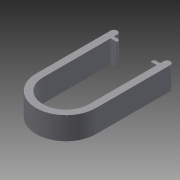
# Autodesk Inventor part: Pinza tapón tornillo
Saved by Autodesk Inventor 2014 (Build 180170000, 170)
## iProperties
Created: 2015-05-28
Part Number: Pinza tapón tornillo
Material: Generic
Document SubType Name: Modeling
Designer: Rubén
Density: 1 g/cm^3
Appearance: Default
Author: Rubén
Autodesk Inventor part; units mm, degrees
ref_plane "YZ Plane" through (0, 0, 0) normal (1, 0, 0) x (0, 1, 0)
ref_plane "XZ Plane" through (0, 0, 0) normal (0, 1, 0) x (-1, 0, 0)
ref_plane "XY Plane" through (0, 0, 0) normal (0, 0, 1) x (1, 0, 0)
sketch "Sketch1" plane through (0, 0, 0) normal (0, 1, 0) x (-1, 0, 0)
  line L0 (10.25, 0) -> (10.25, 30)
  arc A0 (10.25, 30) -> (0, 40.25) centre (0, 30) ccw
  arc A1 (13.25, 30) -> (0, 43.25) centre (0, 30) ccw
  line L1 (13.25, 30) -> (13.25, 0)
  line L2 (0, 0) -> (0, 30) construction
  line L3 (0, 30) -> (13.25, 30) construction
  line L4 (0, 43.25) -> (0, 40.25)
  line L5 (10.25, 0) -> (13.25, 0)
  dimension "d0" = 10.25
  dimension "d1" = 3
  dimension "d2" = 30
  dimension "d3" = 0
  dimension "d4" = 0
  constraints: 12 end point, 4 point on circle, 3 perpendicular, 2 centre point, 2 parallel, 2 tangent, 1 coincident, 1 vertical
  measures "d0" distance between parallel lines of L0 L2
  measures "d1" distance between parallel lines of L1 L0
  measures "d2" distance from line of L2.start L3
  measures "d3" distance between parallel lines of L2 L4
  measures "d4" distance from line of L2.start L5
extrude "Extrusion1" add sketch "Sketch1" along normal blind 10
sketch "Sketch4" plane through (-10.25, 0, 0) normal (0, 0, -1) x (-1, 0, 0)
  line L0 (3, 0) -> (0, 0) projected
  line L1 (3, 0) -> (3, 10) projected
  line L2 (0, 10) -> (3, 10) projected
  line L3 (0, 0) -> (0, 10) projected
  line L4 (0, 10) -> (-2.75, 10)
  line L5 (-2.75, 10) -> (-2.75, 0)
  line L6 (-2.75, 0) -> (0, 0)
  point P0 (-10.25, 0)
  dimension "d13" = 2.75
  constraints: 6 end point, 2 perpendicular, 1 parallel
  measures "d13" distance of L2.start L4.end
extrude "Extrusion3" add sketch "Sketch4" along normal blind 1.5
sketch "Sketch5" plane through (-10.25, 0, -1.5) normal (0, 0, -1) x (-1, 0, 0)
  line L0 (3, 10) -> (-2.75, 10) projected
  line L1 (-2.75, 0) -> (3, 0) projected
  line L2 (3, 0) -> (3, 10) projected
  line L3 (0, 10) -> (0, 0)
  point P0 (-10.25, 0)
  dimension "d16" = 3
  constraints: 2 end point, 2 point on line, 1 perpendicular
  measures "d16" distance between parallel lines of L2 L3
extrude "Extrusion4" add sketch "Sketch5" along normal blind 3
fillet "Fillet1" radius 1.5 2 edges at (-10.25, 5, -4.5) (-13.25, 5, -4.5)
fillet "Fillet2" radius 1 1 edges at (-7.5, 5, -1.5)
mirror "Mirror1" about plane through (0, 0, 43.25) normal (1, 0, 0)
body "Solid1"
